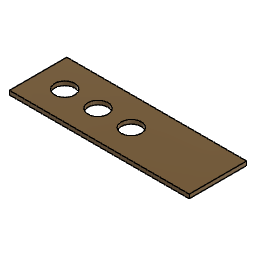
control_panel_top (Autodesk Fusion 360 design; units mm, degrees)
Autodesk Fusion 360 part; units mm, degrees
sketch "Control Panel Top" plane through (0, 0, 0) normal (0, 0, 1) x (1, 0, 0)
  line L0 (0, 0) -> (270, 0)
  line L1 (270, 0) -> (270, 86.085)
  line L2 (270, 86.085) -> (0, 86.085)
  line L3 (0, 86.085) -> (0, 0)
  dimension "d6" = 270
  dimension "d7" = 86.085
  constraint horizontal L0
  constraint vertical L1
  constraint horizontal L2
  constraint vertical L3
  constraint coincident L0.start L3.end
  measures "d6" distance of L0.start L0.end
  measures "d7" distance of L0.end L1.end
extrude "Extrude1" add sketch "Control Panel Top" along normal blind 6
sketch "Button Layout" plane through (0, 0, 6) normal (0, 0, 1) x (-1, 0, 0)
  line L0 (0, -86.085) -> (0, 0)
  line L1 (0, 0) -> (-270, 0)
  line L2 (-270, 0) -> (-270, -86.085)
  line L3 (-270, -86.085) -> (0, -86.085)
  circle A0 centre (-90, -43) radius 15
  circle A1 centre (-140, -43) radius 15
  circle A2 centre (-40, -43) radius 15
  dimension "d12" = 30
  dimension "d13" = 30
  dimension "d14" = 30
  dimension "d17" = 40
  dimension "d20" = 50
  dimension "d21" = 43
  dimension "d22" = 43
  dimension "d23" = 43
  dimension "d24" = 50
  measures "d12" diameter of A0
  measures "d13" diameter of A1
  measures "d14" diameter of A2
  measures "d17" distance of L0 A2.centre
  measures "d20" horizontal distance of A0.centre A1.centre
  measures "d21" distance of L1 A2.centre
  measures "d22" distance of L1 A0.centre
  measures "d23" distance of L1 A1.centre
  measures "d24" distance of A0.centre A2.centre
extrude "Extrude2" cut sketch "Button Layout" against normal blind 6 contours A0 | A1
extrude "Extrude3" cut sketch "Button Layout" against normal blind 6 contours A2
equation "MDFThickness = 6 mm" comment "Thickness of the MDF board"
equation "d2 = MDFThickness"
equation "controlPanelTopLength = 75 mm" comment "Length of the top plate of the control panel"
equation "controlPanelTopWidth = 250 mm" comment "Width of the top plate of the control panel"
equation "d9 = -MDFThickness"
equation "arcadeButtonDiameter = 30 mm" comment "Diameter of the Arcade Game Buttons"
equation "d12 = arcadeButtonDiameter"
equation "d13 = arcadeButtonDiameter"
equation "d14 = arcadeButtonDiameter"
equation "d15 = -MDFThickness"
equation "d21 = ( 86 / 2 ) * 1 mm"
equation "d22 = ( 86 / 2 ) * 1 mm"
equation "d23 = ( 86 / 2 ) * 1 mm"
named bodies: "Control Panel Top"
